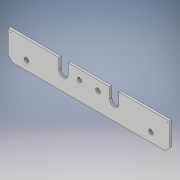
# Autodesk Inventor part: Lauren's Part
Saved by Autodesk Inventor 2017 (Build 210142000, 142)
## iProperties
Created: 2017-05-20
Part Number: Lauren's Part
Material: Generic
Document SubType Name: Modeling
Designer: User
Density: 1 g/cm^3
Appearance: Default
Author: User
Autodesk Inventor part; units mm, degrees
ref_plane "YZ Plane" through (0, 0, 0) normal (1, 0, 0) x (0, 1, 0)
ref_plane "XZ Plane" through (0, 0, 0) normal (0, 1, 0) x (-1, 0, 0)
ref_plane "XY Plane" through (0, 0, 0) normal (0, 0, 1) x (1, 0, 0)
sketch "Sketch1" plane through (0, 0, 0) normal (0, 0, 1) x (1, 0, 0)
  line L0 (0, 0) -> (444.5, 0)
  line L1 (444.5, 0) -> (444.5, 76.2)
  line L2 (444.5, 76.2) -> (0, 76.2)
  line L3 (0, 76.2) -> (0, 0)
  dimension "d0" = 444.5
  dimension "d1" = 76.2
  constraints: 8 end point, 2 parallel, 1 horizontal, 1 perpendicular
  measures "d0" distance of L2.end L1.end
  measures "d1" distance of L1.end L0.end
extrude "Extrusion1" add sketch "Sketch1" along normal blind 6.35
chamfer "Chamfer1" distance 12.7 angle 45 1 edges at (444.5, 0, 3.175)
chamfer "Chamfer2" distance 12.7 angle 45 1 edges at (0, 0, 3.175)
sketch "Sketch2" plane through (0, 0, 6.35) normal (0, 0, 1) x (1, 0, 0)
  line L0 (0, 46.8514) -> (152.4, 46.8514)
  line L1 (444.5, 12.7) -> (444.5, 76.2) projected
  line L2 (292.1, 46.8514) -> (444.5, 46.8514)
  circle A0 centre (152.4, 46.8514) radius 12.7
  circle A1 centre (292.1, 46.8514) radius 12.7
  point P0 (0, 0)
  point P1 (139.7, 46.8514)
  point P2 (165.1, 46.8514)
  dimension "d10" = 152.4
  dimension "d11" = 25.4
  dimension "d12" = 25.4
  constraints: 4 coincident, 4 end point, 2 centre point, 2 point on circle, 1 horizontal, 1 perpendicular, 1 point on line
  measures "d10" distance of L0.start L0.end
  measures "d11" diameter of A0
  measures "d12" diameter of A1
extrude "Extrusion2" cut sketch "Sketch2" against normal blind 25.4
sketch "Sketch3" plane through (0, 0, 6.35) normal (0, 0, 1) x (1, 0, 0)
  circle A0 centre (152.4, 46.8514) radius 12.7 projected
  line L0 (139.7, 46.8514) -> (139.7, 76.2)
  line L1 (165.1, 46.8514) -> (165.1, 76.2)
  line L2 (444.5, 76.2) -> (0, 76.2) projected
  line L3 (139.7, 76.2) -> (165.1, 76.2)
  arc A1 (139.7, 46.8514) -> (165.1, 46.8514) centre (152.4, 46.8514) ccw
  point P0 (0, 0)
  constraints: 6 end point, 5 point on circle, 3 tangent, 2 vertical, 1 centre point, 1 collinear, 1 point on line
extrude "Extrusion3" cut sketch "Sketch3" against normal blind 25.4 contours A0 L0 L2 L1
sketch "Sketch4" plane through (0, 0, 6.35) normal (0, 0, 1) x (1, 0, 0)
  circle A0 centre (292.1, 46.8514) radius 12.7 projected
  line L0 (279.4, 46.8514) -> (279.4, 76.2)
  line L1 (444.5, 76.2) -> (165.1, 76.2) projected
  line L2 (304.8, 46.8514) -> (304.8, 76.2)
  line L3 (304.8, 76.2) -> (279.4, 76.2)
  arc A1 (279.4, 46.8514) -> (304.8, 46.8514) centre (292.1, 46.8514) ccw
  point P0 (0, 0)
  constraints: 6 end point, 2 point on circle, 2 tangent, 1 centre point, 1 collinear, 1 horizontal alignment, 1 midpoint, 1 point on line, 1 vertical, 1 other
extrude "Extrusion4" cut sketch "Sketch4" against normal blind 25.4 contours A0 L0 L1 L2
sketch "Sketch5" plane through (0, 0, 6.35) normal (0, 0, 1) x (1, 0, 0)
  line L0 (0, 76.2) -> (0, 12.7) projected
  line L1 (12.7, 0) -> (431.8, 0) projected
  line L2 (444.5, 12.7) -> (444.5, 76.2) projected
  circle A0 centre (50.8, 25.4) radius 6.35
  circle A1 centre (393.7, 25.4) radius 6.35
  point P0 (0, 0)
  dimension "d19" = 50.8
  dimension "d20" = 25.4
  dimension "d21" = 25.4
  dimension "d22" = 50.8
  dimension "d23" = 12.7
  dimension "d24" = 12.7
  constraints: 2 centre point, 2 coincident
  measures "d19" distance from line of L0 point (50.8, 25.4)
  measures "d20" distance from line of L1 point (50.8, 25.4)
  measures "d21" distance from line of L1 point (393.7, 25.4)
  measures "d22" distance from line of L2 point (393.7, 25.4)
  measures "d23" diameter of A0
  measures "d24" diameter of A1
extrude "Extrusion5" cut sketch "Sketch5" against normal blind 25.4
sketch "Sketch6" plane through (0, 0, 6.35) normal (0, 0, 1) x (1, 0, 0)
  line L0 (139.7, 76.2) -> (0, 76.2) projected
  line L1 (0, 76.2) -> (0, 12.7) projected
  line L2 (444.5, 76.2) -> (304.8, 76.2) projected
  line L3 (444.5, 12.7) -> (444.5, 76.2) projected
  circle A0 centre (6.35, 69.85) radius 0.635
  circle A1 centre (438.15, 69.85) radius 0.635
  point P0 (0, 0)
  dimension "d27" = 6.35
  dimension "d28" = 6.35
  dimension "d29" = 6.35
  dimension "d30" = 6.35
  dimension "d31" = 1.27
  dimension "d32" = 1.27
  constraints: 2 centre point, 2 coincident
  measures "d27" distance from line of point (6.35, 69.85) L0
  measures "d28" distance from line of L1 point (6.35, 69.85)
  measures "d29" distance from line of L2 point (438.15, 69.85)
  measures "d30" distance from line of L3 point (438.15, 69.85)
  measures "d31" diameter of A0
  measures "d32" diameter of A1
extrude "Extrusion6" cut sketch "Sketch6" against normal blind 25.4
sketch "Sketch7" plane through (0, 0, 6.35) normal (0, 0, 1) x (1, 0, 0)
  line L0 (279.4, 76.2) -> (165.1, 76.2) projected
  line L1 (165.1, 76.2) -> (165.1, 46.8514) projected
  line L2 (279.4, 46.8514) -> (279.4, 76.2) projected
  circle A0 centre (196.85, 50.8) radius 6.35
  circle A1 centre (247.65, 50.8) radius 6.35
  point P0 (0, 0)
  dimension "d35" = 25.4
  dimension "d36" = 31.75
  dimension "d37" = 25.4
  dimension "d38" = 31.75
  dimension "d39" = 12.7
  dimension "d40" = 12.7
  constraints: 2 centre point, 2 coincident
  measures "d35" distance from line of L0 point (196.85, 50.8)
  measures "d36" distance from line of L1 point (196.85, 50.8)
  measures "d37" distance from line of L0 point (247.65, 50.8)
  measures "d38" distance from line of L2 point (247.65, 50.8)
  measures "d39" diameter of A0
  measures "d40" diameter of A1
extrude "Extrusion7" cut sketch "Sketch7" against normal blind 25.4
body "Solid1"
